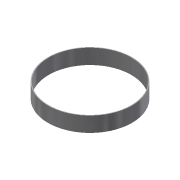
# Autodesk Inventor part: PP-03
Saved by Autodesk Inventor 2022 (Build 260148000, 148)
## iProperties
Created: 2008-09-23
Part Number: PP-03
Document SubType Name: Modeling
Designer: Mark Flayler
Mass: 0.0246534 g
Surface Area: 0.825962 cm^2
Volume: 0.00313657 cm^3
Density: 7.86 g/cm^3
Material: Steel, Mild
Description: RING
Appearance: Steel
Author: Mark Flayler
Autodesk Inventor part; units mm, degrees
ref_plane "YZ Plane" through (0, 0, 0) normal (1, 0, 0) x (0, 1, 0)
ref_plane "XZ Plane" through (0, 0, 0) normal (0, 1, 0) x (-1, 0, 0)
ref_plane "XY Plane" through (0, 0, 0) normal (0, 0, 1) x (1, 0, 0)
sketch "Sketch1" plane through (0, 0, 0) normal (0, 0, 1) x (1, 0, 0)
  circle A0 centre (0, 0) radius 4.2
  circle A1 centre (0, 0) radius 4.12
  dimension "d0" = 8.4
  dimension "d1" = 8.24
  constraints: 2 centre point, 2 coincident
  measures "d0" diameter of A0
  measures "d1" diameter of A1
extrude "Extrusion1" add sketch "Sketch1" along normal blind 1.5
body "Solid1"
